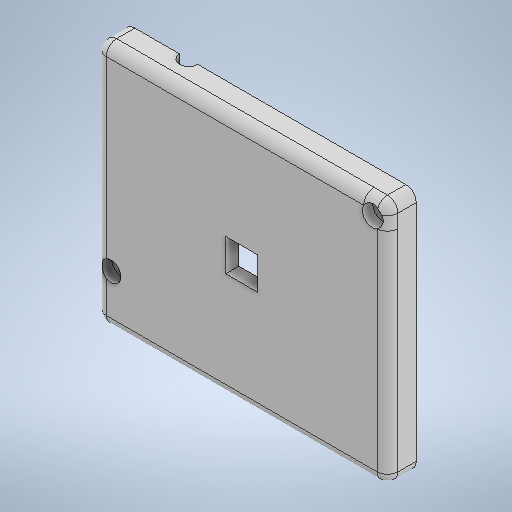
# Autodesk Inventor part: Lid
Saved by Autodesk Inventor 2025.2 (Build 292293000, 293)
## iProperties
Created: 2025-01-26
Part Number: Lid
Material: Generisch
Document SubType Name: Modeling
Designer: Envy
Density: 1 g/cm^3
Appearance: Vorgabe
Author: Envy
Autodesk Inventor part; units mm, degrees
ref_plane "YZ Plane" through (0, 0, 0) normal (1, 0, 0) x (0, 1, 0)
ref_plane "XZ Plane" through (0, 0, 0) normal (0, 1, 0) x (-1, 0, 0)
ref_plane "Arbeitsebene1" through (26, 12.1004, 0) normal (0, 0, 1) x (1, 0, 0)
sketch "Skizze1" plane through (26, 12.1004, 0) normal (0, 0, 1) x (1, 0, 0)
  arc A0 (-54, -33.6004) -> (-52, -35.6004) centre (-52, -33.6004) ccw projected
  line L0 (-52, -35.6004) -> (0, -35.6004) projected
  arc A1 (0, -35.6004) -> (2, -33.6004) centre (0, -33.6004) ccw projected
  line L1 (2, -33.6004) -> (2, 9.3996) projected
  arc A2 (2, 9.3996) -> (0, 11.3996) centre (0, 9.3996) ccw projected
  line L2 (0, 11.3996) -> (-52, 11.3996) projected
  arc A3 (-52, 11.3996) -> (-54, 9.3996) centre (-52, 9.3996) ccw projected
  line L3 (-54, 9.3996) -> (-54, -33.6004) projected
  circle A4 centre (-0.95, 8.4496) radius 0.95 projected
  circle A5 centre (-51.05, -25.8004) radius 0.95 projected
  arc A6 (-24.2441, 3.8663) -> (-23.5, 4.8331) centre (-24.5, 4.8331) ccw projected
  line L4 (-23.5, 5.8996) -> (-23.5, 4.8331) projected
  line L5 (-24.5, 5.8996) -> (-23.5, 5.8996) projected
  line L6 (-24.5, 9.3996) -> (-24.5, 5.8996) projected
  line L7 (-24.5, 9.3996) -> (-7.5, 9.3996) projected
  line L8 (-7.5, 5.8996) -> (-7.5, 9.3996) projected
  line L9 (-8.5, 5.8996) -> (-7.5, 5.8996) projected
  line L10 (-8.5, 4.8996) -> (-8.5, 5.8996) projected
  arc A7 (-8.5, 4.8996) -> (-7.5, 3.8996) centre (-7.5, 4.8996) ccw projected
  line L11 (-7, 3.8996) -> (-7.5, 3.8996) projected
  arc A8 (-7, 3.8996) -> (-6, 4.8996) centre (-7, 4.8996) ccw projected
  line L12 (-6, 9.3996) -> (-6, 4.8996) projected
  line L13 (-6, 9.3996) -> (-4.3996, 9.3996) projected
  arc A9 (-3.3997, 8.4141) -> (-4.3996, 9.3996) centre (-4.3996, 8.3996) ccw projected
  arc A10 (-3.3997, 8.4141) -> (-0.9855, 5.9999) centre (-0.95, 8.4496) ccw projected
  arc A11 (0, 5) -> (-0.9855, 5.9999) centre (-1, 5) ccw projected
  line L14 (0, 5) -> (0, -25.7504) projected
  arc A12 (-0.5, -26.6164) -> (0, -25.7504) centre (-1, -25.7504) ccw projected
  arc A13 (-0.5, -26.6164) -> (-1, -27.4824) centre (0, -27.4824) ccw projected
  line L15 (-1, -28.7504) -> (-1, -27.4824) projected
  line L16 (0, -28.7504) -> (-1, -28.7504) projected
  line L17 (0, -28.7504) -> (0, -33.6004) projected
  line L18 (0, -33.6004) -> (-52, -33.6004) projected
  line L19 (-52, -33.6004) -> (-52, -28.7504) projected
  line L20 (-51, -28.7504) -> (-52, -28.7504) projected
  line L21 (-51, -28.6986) -> (-51, -28.7504) projected
  arc A14 (-50.5932, -28.2074) -> (-51, -28.6986) centre (-50.5, -28.6986) ccw projected
  arc A15 (-50.5932, -28.2074) -> (-51.0145, -23.3506) centre (-51.05, -25.8004) ccw projected
  arc A16 (-52, -22.3507) -> (-51.0145, -23.3506) centre (-51, -22.3507) ccw projected
  line L22 (-52, -22.3507) -> (-52, 2.2996) projected
  arc A17 (-51.5, 3.1657) -> (-52, 2.2996) centre (-51, 2.2996) ccw projected
  arc A18 (-51.5, 3.1657) -> (-51, 4.0317) centre (-52, 4.0317) ccw projected
  line L23 (-51, 5.2996) -> (-51, 4.0317) projected
  line L24 (-52, 5.2996) -> (-51, 5.2996) projected
  line L25 (-52, 5.2996) -> (-52, 9.3996) projected
  line L26 (-52, 9.3996) -> (-26, 9.3996) projected
  line L27 (-26, 5.2996) -> (-26, 9.3996) projected
  line L28 (-27, 5.2996) -> (-26, 5.2996) projected
  line L29 (-27, 4.2996) -> (-27, 5.2996) projected
  arc A19 (-27, 4.2996) -> (-26, 3.2996) centre (-26, 4.2996) ccw projected
  line L30 (-25.4165, 3.2996) -> (-26, 3.2996) projected
  arc A20 (-25.4165, 3.2996) -> (-24.7024, 3.5996) centre (-25.4165, 4.2996) ccw projected
  arc A21 (-24.2441, 3.8663) -> (-24.7024, 3.5996) centre (-23.9882, 2.8996) ccw projected
  point P0 (-26, -12.1004)
extrude "Extrusion1" add sketch "Skizze1" along normal blind 2.5 contours L3 A3 L2 A2 L1 A1 L0 A0 | A6 L4 L5 L6 L7 L8 L9 L10 A7 L11 A8 L12 L13 A9 A10 A11 L14 A12 A13 L15 L16 L17 L18 L19 L20 L21 A14 A15 A16 L22 A17 A18 L23 L24 L25 L26 L27 L28 L29 A19 L30 A20 A21
sketch "Skizze2" plane through (26, 12.1004, 2.5) normal (0, 0, 1) x (1, 0, 0)
  circle A0 centre (-0.95, 8.4496) radius 0.95 projected
  circle A1 centre (-51.05, -25.8004) radius 0.95 projected
  circle A2 centre (-51.05, -25.8004) radius 1.9
  circle A3 centre (-0.95, 8.4496) radius 1.9
  point P0 (-26, -12.1004)
  dimension "d2" = 3.8
  dimension "d3" = 3.8
  constraints: 2 centre point, 2 coincident
  measures "d2" diameter of A2
  measures "d3" diameter of A3
extrude "Extrusion2" cut sketch "Skizze2" against normal blind 2
fillet "Rundung1" radius 1.99 8 edges at (27.4142, 22.9142, 2.5) (0, 23.5, 2.5) (-27.4142, 22.9142, 2.5) (-28, 0, 2.5) (-27.4142, -22.9142, 2.5) (0, -23.5, 2.5) (27.4142, -22.9142, 2.5) (28, 0, 2.5)
sketch "Skizze3" plane through (26, 12.1004, 2.5) normal (0, 0, 1) x (1, 0, 0)
  line L0 (-22.95, -9.0004) -> (-29.05, -9.0004)
  line L1 (-29.05, -9.0004) -> (-29.05, -15.2004)
  line L2 (-29.05, -15.2004) -> (-22.95, -15.2004)
  line L3 (-22.95, -15.2004) -> (-22.95, -9.0004)
  line L4 (-22.95, -9.0004) -> (-29.05, -15.2004) construction
  line L5 (-29.05, -9.0004) -> (-22.95, -15.2004) construction
  point P0 (-26, -12.1004)
  dimension "d7" = 6.1
  dimension "d8" = 6.2
  constraints: 12 end point, 2 midpoint, 2 parallel, 1 horizontal, 1 perpendicular
  measures "d7" distance of L2.end L1.end
  measures "d8" distance of L1.end L0.end
extrude "Extrusion3" cut sketch "Skizze3" against normal through all
sketch "Skizze5" plane through (26, 12.1004, 0) normal (0, 0, -1) x (-1, 0, 0)
  line L0 (0, 9.3996) -> (52, 9.3996)
  line L1 (52, 9.3996) -> (52, -33.6004)
  line L2 (52, -33.6004) -> (0, -33.6004)
  line L3 (0, -33.6004) -> (0, 9.3996)
  line L4 (0, 11.3996) -> (52, 11.3996) projected
  line L5 (52, -35.6004) -> (0, -35.6004) projected
  line L6 (54, 9.3996) -> (54, -33.6004) projected
  line L7 (-2, -33.6004) -> (-2, 9.3996) projected
  line L8 (29.05, -15.2004) -> (22.95, -15.2004) projected
  line L9 (22.95, -15.2004) -> (22.95, -9.0004) projected
  line L10 (22.95, -9.0004) -> (29.05, -9.0004) projected
  line L11 (29.05, -9.0004) -> (29.05, -15.2004) projected
  line L12 (52, -35.6004) -> (0, -35.6004) projected
  arc A0 (52, -35.6004) -> (54, -33.6004) centre (52, -33.6004) ccw projected
  line L13 (54, 9.3996) -> (54, -33.6004) projected
  arc A1 (54, 9.3996) -> (52, 11.3996) centre (52, 9.3996) ccw projected
  line L14 (0, 11.3996) -> (52, 11.3996) projected
  arc A2 (0, 11.3996) -> (-2, 9.3996) centre (0, 9.3996) ccw projected
  line L15 (-2, -33.6004) -> (-2, 9.3996) projected
  arc A3 (-2, -33.6004) -> (0, -35.6004) centre (0, -33.6004) ccw projected
  circle A4 centre (0.95, 8.4496) radius 0.95 projected
  circle A5 centre (51.05, -25.8004) radius 0.95 projected
  point P0 (26, -12.1004)
  point P1 (54, -33.6004)
  point P2 (54, 9.3996)
  point P3 (52, 11.3996)
  point P4 (0, 11.3996)
  point P5 (-2, 9.3996)
  point P6 (-2, -33.6004)
  point P7 (0, -35.6004)
  dimension "d11" = 2
  dimension "d12" = 2
  dimension "d13" = 2
  dimension "d14" = 2
  constraints: 8 end point, 2 parallel, 1 horizontal, 1 perpendicular
  measures "d11" distance between parallel lines of L0 L4
  measures "d12" distance between parallel lines of L5 L2
  measures "d13" distance between parallel lines of L6 L1
  measures "d14" distance between parallel lines of L7 L3
extrude "Extrusion4" add sketch "Skizze5" along normal blind 3 contours L4 A1 L6 A0 L5 A3 L7 A2
sketch "Skizze6" plane through (-26, 23.5, 0.51) normal (0, 1, 0) x (1, 0, 0)
  line L0 (52, 3.51) -> (0, 3.51) projected
  circle A0 centre (10.3315, 3.51) radius 1.75
  point P0 (26, 0.51)
  point P1 (8.5815, 3.51)
  point P2 (12.0815, 3.51)
  dimension "d17" = 3.5
  constraints: 1 centre point, 1 point on line
  measures "d17" diameter of A0
extrude "Extrusion5" cut sketch "Skizze6" against normal blind 3 contours A0 L0 picked at (10.0001, 3.0299)
sketch "Skizze7" plane through (26, 12.1004, 0) normal (0, 0, -1) x (-1, 0, 0)
  line L0 (29.05, -15.2004) -> (22.95, -15.2004) projected
  line L1 (22.95, -15.2004) -> (22.95, -9.0004) projected
  line L2 (22.95, -9.0004) -> (29.05, -9.0004) projected
  line L3 (29.05, -9.0004) -> (29.05, -15.2004) projected
  line L4 (52, 9.3996) -> (0.95, 9.3996) projected
  arc A0 (0, 8.4496) -> (0.95, 9.3996) centre (0.95, 8.4496) ccw projected
  line L5 (0, 8.4496) -> (0, -33.6004) projected
  line L6 (0, -33.6004) -> (52, -33.6004) projected
  line L7 (52, -33.6004) -> (52, -25.8004) projected
  circle A1 centre (51.05, -25.8004) radius 0.95 projected
  line L8 (52, -25.8004) -> (52, 9.3996) projected
  circle A2 centre (51.05, -25.8004) radius 2.45
  circle A3 centre (0.95, 8.4496) radius 2.45
  line L9 (39.9185, 9.3996) -> (39.9185, 11.3996) projected
  line L10 (39.9185, 11.3996) -> (0, 11.3996) projected
  arc A4 (0, 11.3996) -> (-2, 9.3996) centre (0, 9.3996) ccw projected
  line L11 (-2, 9.3996) -> (-2, -33.6004) projected
  arc A5 (-2, -33.6004) -> (0, -35.6004) centre (0, -33.6004) ccw projected
  line L12 (0, -35.6004) -> (52, -35.6004) projected
  arc A6 (52, -35.6004) -> (54, -33.6004) centre (52, -33.6004) ccw projected
  line L13 (54, -33.6004) -> (54, 9.3996) projected
  arc A7 (54, 9.3996) -> (52, 11.3996) centre (52, 9.3996) ccw projected
  line L14 (52, 11.3996) -> (43.4185, 11.3996) projected
  line L15 (43.4185, 11.3996) -> (43.4185, 9.3996) projected
  line L16 (43.4185, 9.3996) -> (52, 9.3996) projected
  line L17 (52, 9.3996) -> (52, -33.6004) projected
  line L18 (52, -33.6004) -> (0, -33.6004) projected
  line L19 (0, -33.6004) -> (0, 9.3996) projected
  line L20 (0, 9.3996) -> (39.9185, 9.3996) projected
  arc A8 (0.95, 9.3996) -> (0, 8.4496) centre (0.95, 8.4496) ccw projected
  point P0 (26, -12.1004)
  point P1 (52, -23.542)
  point P2 (52, -28.0587)
  point P3 (0.95, 9.3996)
  point P4 (0.95, 9.3996)
  point P5 (0.95, 9.3996)
  point P6 (3.2083, 9.3996)
  point P7 (0, 6.1913)
  dimension "d20" = 1.5
  dimension "d21" = 1.5
  constraints: 2 centre point, 2 coincident, 1 horizontal alignment
  measures "d21" radial gap between concentric circles of A3 A0
extrude "Extrusion6" add sketch "Skizze7" along normal blind 3 contours L8 L7 A2 | A3 L5 A0 L4 | A8 L19 L20 picked at (49.1338, -25.5256)
